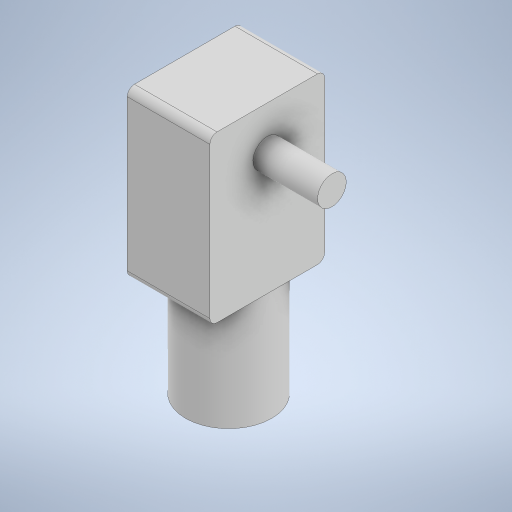
# Autodesk Inventor part: MOTOR 2
Saved by Autodesk Inventor 2024.4 (Build 284460000, 460)
## iProperties
Created: 2025-12-18
Part Number: MOTOR 2
Material: Generic
Document SubType Name: Modeling
Designer: hp
Density: 1 g/cm^3
Appearance: Default
Author: hp
Autodesk Inventor part; units mm, degrees
ref_plane "YZ Plane" through (0, 0, 0) normal (1, 0, 0) x (0, 1, 0)
ref_plane "XZ Plane" through (0, 0, 0) normal (0, 1, 0) x (-1, 0, 0)
ref_plane "XY Plane" through (0, 0, 0) normal (0, 0, 1) x (1, 0, 0)
sketch "Sketch1" plane through (0, 0, 0) normal (1, 0, 0) x (0, 1, 0)
  line L0 (2, 0) -> (44, 0)
  line L1 (46, 2) -> (46, 30)
  line L2 (44, 32) -> (2, 32)
  line L3 (0, 30) -> (0, 2)
  arc A0 (2, 32) -> (0, 30) centre (2, 30) ccw
  arc A1 (46, 30) -> (44, 32) centre (44, 30) ccw
  arc A2 (44, 0) -> (46, 2) centre (44, 2) ccw
  arc A3 (0, 2) -> (2, 0) centre (2, 2) ccw
  line L4 (55.8524, 16) -> (-12.4215, 16) construction
  circle A4 centre (33.9212, 16) radius 4
  point P0 (0, 0)
  dimension "d3" = 8
  constraints: 10 end point, 8 point on circle, 8 tangent, 5 centre point, 3 equal radius, 3 point on line, 2 horizontal, 2 parallel, 1 perpendicular
  measures "d3" diameter of A4
extrude "Extrusion1" add sketch "Sketch1" along normal blind 23
extrude "Extrusion2" add sketch "Sketch1" along normal blind 41 contours A4
sketch "Sketch2" plane through (0, 0, 2) normal (0, -1, 0) x (1, 0, 0)
  line L0 (41, 10) -> (41, 18) projected
  line L1 (41, 14) -> (-14.7387, 14) construction
  circle A0 centre (10.7172, 12.4863) radius 12
  point P0 (0, -2)
  dimension "d12" = 24
  constraints: 2 end point, 1 centre point, 1 horizontal, 1 midpoint
  measures "d12" diameter of A0
extrude "Extrusion3" add sketch "Sketch2" along normal blind 31
body "Solid1"
